# Autodesk Inventor part: SYNC_SJ
Saved by Autodesk Inventor 2016 (Build 200138000, 138)
## iProperties
Created: 2016-04-08
Part Number: SYNC_SJ
Material: Generic
Document SubType Name: Modeling
Designer: Paschalis
Density: 1 g/cm^3
Appearance: SJ, SYNC_SJ
Author: Paschalis
Autodesk Inventor part; units mm, degrees
ref_plane "YZ Plane" through (0, 0, 0) normal (1, 0, 0) x (0, 1, 0)
ref_plane "XZ Plane" through (0, 0, 0) normal (0, 1, 0) x (-1, 0, 0)
ref_plane "XY Plane" through (0, 0, 0) normal (0, 0, 1) x (1, 0, 0)
sketch "SJ, SYNC_SJ_121" plane through (0, 0, 0) normal (0, 0, 1) x (1, 0, 0)
  line L0 (-1.651, 1.016) -> (1.651, 1.016)
  line L1 (1.651, 1.016) -> (1.651, -1.0922)
  line L2 (1.651, -1.0922) -> (-1.651, -1.0922)
  line L3 (-1.651, -1.0922) -> (-1.651, 1.016)
  constraints: 8 end point
extrude "Extrusion1" add sketch "SJ, SYNC_SJ_121" along normal blind 1
body "Solid1"
